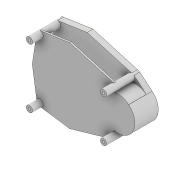
# Autodesk Inventor part: base
Saved by Autodesk Inventor 2020 (Build 240168000, 168)
## iProperties
Created: 2020-08-31
Part Number: base
Material: 일반
Document SubType Name: Modeling
Designer: 이호석
Mass: 51.1495 g
Surface Area: 251.219 cm^2
Volume: 51.1495 cm^3
Density: 1 g/cm^3
Appearance: 기본값
Author: 이호석
Autodesk Inventor part; units mm, degrees
ref_plane "YZ Plane" through (0, 0, 0) normal (1, 0, 0) x (0, 1, 0)
ref_plane "XZ Plane" through (0, 0, 0) normal (0, 1, 0) x (-1, 0, 0)
ref_plane "XY Plane" through (0, 0, 0) normal (0, 0, 1) x (1, 0, 0)
sketch "스케치1" plane through (0, 0, 0) normal (0, 0, 1) x (1, 0, 0)
  line L0 (0, 0) -> (-35.14, 0)
  line L1 (-35.14, 0) -> (61.6, 0)
  line L2 (0, 35.14) -> (0, -35.14)
  line L3 (-35.14, -35.14) -> (61.6, -35.14)
  line L4 (61.6, -35.14) -> (61.6, 35.14)
  line L5 (61.6, 35.14) -> (-35.14, 35.14)
  line L6 (-35.14, 35.14) -> (-35.14, -35.14)
  line L7 (0, 0) -> (-27.87, 0)
  line L8 (0, 0) -> (42, 0)
  line L9 (42, 20) -> (42, -20)
  circle A0 centre (42, -20) radius 1.25
  circle A1 centre (42, 20) radius 1.25
  line L10 (0, 0) -> (45.5, 0)
  circle A2 centre (45.5, 0) radius 9
  circle A3 centre (45.5, 0) radius 16.1
  circle A4 centre (42, -20) radius 3
  circle A5 centre (42, 20) radius 3
  line L11 (45.5, 0) -> (61.6, 0) construction
  line L12 (42, 20) -> (45, 20) construction
  line L13 (44.1213, 22.1213) -> (55.8489, 12.3333)
  line L14 (42, 23) -> (0, 35.14)
  line L15 (-27.87, 28) -> (-27.87, -28)
  circle A6 centre (-27.87, 28) radius 1.25
  circle A7 centre (-27.87, 28) radius 3
  circle A8 centre (-27.87, -28) radius 1.25
  circle A9 centre (-27.87, -28) radius 3
  line L16 (-27.87, 31) -> (0, 35.14)
  line L17 (-30.87, 28) -> (-35.14, 0)
  line L18 (44.1213, -22.1213) -> (55.8489, -12.3333)
  line L19 (42, -23) -> (0, -35.14)
  line L20 (-27.87, -31) -> (0, -35.14)
  line L21 (-30.87, -28) -> (-35.14, 0)
  dimension "d20" = 6
  dimension "d0" = 35.14
  dimension "d1" = 96.74
  dimension "d3" = 70.28
  dimension "d4" = 27.87
  dimension "d9" = 42
  dimension "d11" = 40
  dimension "d12" = 2.5
  dimension "d13" = 2.5
  dimension "d14" = 45.5
  dimension "d15" = 18
  dimension "d16" = 32.2
  dimension "d19" = 6
  dimension "d27" = 56
  dimension "d28" = 2.5
  dimension "d29" = 6
  dimension "d30" = 2.5
  dimension "d31" = 6
  constraints: 44 end point, 10 coincident, 9 centre point, 7 symmetric about line, 5 point on line, 4 horizontal, 4 point on circle, 2 parallel, 1 perpendicular, 3 other
  measures "d0" distance of L0.start L0.end
  measures "d1" distance of L0.end L1.end
  measures "d3" distance of L2.start L2.end
  measures "d4" distance of L0.start L7.end
  measures "d9" distance of L0.start L8.end
  measures "d11" distance of L9.start L9.end
  measures "d12" diameter of A0
  measures "d13" diameter of A1
  measures "d14" distance of L0.start L10.end
  measures "d15" diameter of A2
  measures "d16" diameter of A3
  measures "d19" diameter of A4
  measures "d27" distance of L15.start L15.end
  measures "d28" diameter of A6
  measures "d29" diameter of A7
  measures "d30" diameter of A8
  measures "d31" diameter of A9
extrude "돌출1" add sketch "스케치1" along normal blind 5.5 contours L2 L20 A9 L15 L0 | L2 L14 A5 L9 A3 L1 | L0 L15 A7 L16 L2 | L1 A3 L9 A4 L19 L2 | L15 A9 L21 L0 | L0 L17 A7 L15 | A3 L9 A2 L1 | L1 A2 L9 A3 | A7 | A9 | A2 L9 L1 | L1 L9 A2 | A3 L1 A2 L9 | L9 A5 L13 A3 | A3 L18 A4 L9 | L9 A2 L1 A3 | A5 | A4 | L9 A2 L1 | L1 A2 L9
sketch "스케치2" plane through (0, 0, 5.5) normal (0, 0, 1) x (1, 0, 0)
  line L0 (0, 0) -> (-35.14, 0)
  line L1 (-35.14, 0) -> (61.6, 0)
  line L2 (0, 35.14) -> (0, -35.14)
  line L3 (-35.14, -35.14) -> (61.6, -35.14)
  line L4 (61.6, -35.14) -> (61.6, 35.14)
  line L5 (61.6, 35.14) -> (-35.14, 35.14)
  line L6 (-35.14, 35.14) -> (-35.14, -35.14)
  line L7 (0, 0) -> (-27.87, 0)
  line L8 (0, 0) -> (42, 0)
  line L9 (42, 20) -> (42, -20)
  circle A0 centre (42, -20) radius 1.25
  circle A1 centre (42, 20) radius 1.25
  line L10 (0, 0) -> (45.5, 0)
  circle A2 centre (45.5, 0) radius 9
  circle A3 centre (45.5, 0) radius 16.1
  circle A4 centre (42, -20) radius 3
  circle A5 centre (42, 20) radius 3
  line L11 (45.5, 0) -> (61.6, 0) construction
  line L12 (42, 20) -> (45, 20) construction
  line L13 (44.1213, 22.1213) -> (55.8489, 12.3333)
  line L14 (42, 23) -> (0, 35.14)
  line L15 (-27.87, 28) -> (-27.87, -28)
  circle A6 centre (-27.87, 28) radius 1.25
  circle A7 centre (-27.87, 28) radius 3
  circle A8 centre (-27.87, -28) radius 1.25
  circle A9 centre (-27.87, -28) radius 3
  line L16 (-27.87, 31) -> (0, 35.14)
  line L17 (-30.87, 28) -> (-35.14, 0)
  line L18 (-27.87, -31) -> (0, -35.14)
  line L19 (-30.87, -28) -> (-35.14, 0)
  line L20 (42, -23) -> (0, -35.14)
  line L21 (44.1213, -22.1213) -> (55.8489, -12.3333)
  point P0 (55.7837, -12.3877)
  point P1 (55.7837, 12.3877)
  dimension "d46" = 6
  dimension "d34" = 35.14
  dimension "d35" = 96.74
  dimension "d36" = 70.28
  dimension "d37" = 27.87
  dimension "d38" = 42
  dimension "d39" = 40
  dimension "d40" = 2.5
  dimension "d41" = 2.5
  dimension "d42" = 45.5
  dimension "d43" = 18
  dimension "d44" = 32.2
  dimension "d45" = 6
  dimension "d47" = 56
  dimension "d48" = 2.5
  dimension "d49" = 6
  dimension "d50" = 2.5
  dimension "d51" = 6
  constraints: 44 end point, 10 coincident, 9 centre point, 7 symmetric about line, 5 point on line, 4 horizontal, 4 point on circle, 2 parallel, 1 perpendicular, 1 vertical alignment, 2 other
  measures "d34" distance of L0.start L0.end
  measures "d35" distance of L0.end L1.end
  measures "d36" distance of L2.start L2.end
  measures "d37" distance of L0.start L7.end
  measures "d38" distance of L0.start L8.end
  measures "d39" distance of L9.start L9.end
  measures "d40" diameter of A0
  measures "d41" diameter of A1
  measures "d42" distance of L0.start L10.end
  measures "d43" diameter of A2
  measures "d44" diameter of A3
  measures "d45" diameter of A4
  measures "d47" distance of L15.start L15.end
  measures "d48" diameter of A6
  measures "d49" diameter of A7
  measures "d50" diameter of A8
  measures "d51" diameter of A9
extrude "돌출2" add sketch "스케치2" along normal blind 15 contours A3 L9 A2 L1 | L1 A2 L9 A3 | A7 | A9 | A2 L9 L1 | L1 L9 A2 | A3 L1 A2 L9 | L9 A2 L1 A3 | A5 | A4 | L9 A2 L1 | L1 A2 L9
sketch "스케치3" plane through (0, 0, 20.5) normal (0, 0, 1) x (1, 0, 0)
  line L0 (0, 0) -> (-35.14, 0)
  line L1 (-35.14, 0) -> (61.6, 0)
  line L2 (0, 35.14) -> (0, -35.14)
  line L3 (-35.14, -35.14) -> (61.6, -35.14)
  line L4 (61.6, -35.14) -> (61.6, 35.14)
  line L5 (61.6, 35.14) -> (-35.14, 35.14)
  line L6 (-35.14, 35.14) -> (-35.14, -35.14)
  line L7 (0, 0) -> (-27.87, 0)
  line L8 (0, 0) -> (42, 0)
  line L9 (42, 20) -> (42, -20)
  circle A0 centre (42, -20) radius 1.25
  circle A1 centre (42, 20) radius 1.25
  line L10 (0, 0) -> (45.5, 0)
  circle A2 centre (45.5, 0) radius 9
  circle A3 centre (45.5, 0) radius 16.1
  circle A4 centre (42, -20) radius 3
  circle A5 centre (42, 20) radius 3
  line L11 (45.5, 0) -> (61.6, 0) construction
  line L12 (42, 20) -> (45, 20) construction
  line L13 (44.1213, 22.1213) -> (55.8489, 12.3333)
  line L14 (42, 23) -> (0, 35.14)
  line L15 (-27.87, 28) -> (-27.87, -28)
  circle A6 centre (-27.87, 28) radius 1.25
  circle A7 centre (-27.87, 28) radius 3
  circle A8 centre (-27.87, -28) radius 1.25
  circle A9 centre (-27.87, -28) radius 3
  line L16 (-27.87, 31) -> (0, 35.14)
  line L17 (-30.87, 28) -> (-35.14, 0)
  line L18 (-27.87, -31) -> (0, -35.14)
  line L19 (-30.87, -28) -> (-35.14, 0)
  line L20 (42, -23) -> (0, -35.14)
  line L21 (44.1213, -22.1213) -> (55.8489, -12.3333)
  point P0 (42, -15.715)
  point P1 (55.7837, -12.3877)
  point P2 (55.7837, 12.3877)
  point P3 (42, 15.715)
  point P4 (42, 17)
  point P5 (42, -17)
  dimension "d66" = 6
  dimension "d54" = 35.14
  dimension "d55" = 96.74
  dimension "d56" = 70.28
  dimension "d57" = 27.87
  dimension "d58" = 42
  dimension "d59" = 40
  dimension "d60" = 2.5
  dimension "d61" = 2.5
  dimension "d62" = 45.5
  dimension "d63" = 18
  dimension "d64" = 32.2
  dimension "d65" = 6
  dimension "d67" = 56
  dimension "d68" = 2.5
  dimension "d69" = 6
  dimension "d70" = 2.5
  dimension "d71" = 6
  constraints: 44 end point, 10 coincident, 9 centre point, 7 symmetric about line, 5 point on line, 4 horizontal, 4 point on circle, 2 parallel, 1 perpendicular, 3 other
  measures "d54" distance of L0.start L0.end
  measures "d55" distance of L0.end L1.end
  measures "d56" distance of L2.start L2.end
  measures "d57" distance of L0.start L7.end
  measures "d58" distance of L0.start L8.end
  measures "d59" distance of L9.start L9.end
  measures "d60" diameter of A0
  measures "d61" diameter of A1
  measures "d62" distance of L0.start L10.end
  measures "d63" diameter of A2
  measures "d64" diameter of A3
  measures "d65" diameter of A4
  measures "d67" distance of L15.start L15.end
  measures "d68" diameter of A6
  measures "d69" diameter of A7
  measures "d70" diameter of A8
  measures "d71" diameter of A9
extrude "돌출3" add sketch "스케치3" along normal blind 1.6 contours L2 L18 A9 L15 L0 | L2 L14 A5 L9 A3 L1 | L0 L15 A7 L16 L2 | L1 A3 L9 A4 L20 L2 | L15 A9 L19 L0 | L0 L17 A7 L15 | A3 L9 A2 L1 | L1 A2 L9 A3 | A7 | A9 | A2 L9 L1 | L1 L9 A2 | A3 L1 A2 L9 | L9 A2 L1 A3 | A5 | A4 | L9 A2 L1 | L1 A2 L9
sketch "스케치4" plane through (0, 0, 22.1) normal (0, 0, 1) x (1, 0, 0)
  line L0 (0, 0) -> (-35.14, 0)
  line L1 (-35.14, 0) -> (61.6, 0)
  line L2 (0, 35.14) -> (0, -35.14)
  line L3 (-35.14, -35.14) -> (61.6, -35.14)
  line L4 (61.6, -35.14) -> (61.6, 35.14)
  line L5 (61.6, 35.14) -> (-35.14, 35.14)
  line L6 (-35.14, 35.14) -> (-35.14, -35.14)
  line L7 (0, 0) -> (-27.87, 0)
  line L8 (0, 0) -> (42, 0)
  line L9 (42, 20) -> (42, -20)
  circle A0 centre (42, -20) radius 1.25
  circle A1 centre (42, 20) radius 1.25
  line L10 (0, 0) -> (45.5, 0)
  circle A2 centre (45.5, 0) radius 9
  circle A3 centre (45.5, 0) radius 16.1
  circle A4 centre (42, -20) radius 3
  circle A5 centre (42, 20) radius 3
  line L11 (45.5, 0) -> (61.6, 0) construction
  line L12 (42, 20) -> (45, 20) construction
  line L13 (44.1213, 22.1213) -> (55.8489, 12.3333)
  line L14 (42, 23) -> (0, 35.14)
  line L15 (-27.87, 28) -> (-27.87, -28)
  circle A6 centre (-27.87, 28) radius 1.25
  circle A7 centre (-27.87, 28) radius 3
  circle A8 centre (-27.87, -28) radius 1.25
  circle A9 centre (-27.87, -28) radius 3
  line L16 (-27.87, 31) -> (0, 35.14)
  line L17 (-30.87, 28) -> (-35.14, 0)
  line L18 (-27.87, -31) -> (0, -35.14)
  line L19 (-30.87, -28) -> (-35.14, 0)
  line L20 (42, -23) -> (0, -35.14)
  line L21 (44.1213, -22.1213) -> (55.8489, -12.3333)
  dimension "d86" = 6
  dimension "d74" = 35.14
  dimension "d75" = 96.74
  dimension "d76" = 70.28
  dimension "d77" = 27.87
  dimension "d78" = 42
  dimension "d79" = 40
  dimension "d80" = 2.5
  dimension "d81" = 2.5
  dimension "d82" = 45.5
  dimension "d83" = 18
  dimension "d84" = 32.2
  dimension "d85" = 6
  dimension "d87" = 56
  dimension "d88" = 2.5
  dimension "d89" = 6
  dimension "d90" = 2.5
  dimension "d91" = 6
  constraints: 44 end point, 10 coincident, 9 centre point, 7 symmetric about line, 5 point on line, 4 horizontal, 4 point on circle, 2 parallel, 1 perpendicular, 1 vertical alignment, 2 other
  measures "d74" distance of L0.start L0.end
  measures "d75" distance of L0.end L1.end
  measures "d76" distance of L2.start L2.end
  measures "d77" distance of L0.start L7.end
  measures "d78" distance of L0.start L8.end
  measures "d79" distance of L9.start L9.end
  measures "d80" diameter of A0
  measures "d81" diameter of A1
  measures "d82" distance of L0.start L10.end
  measures "d83" diameter of A2
  measures "d84" diameter of A3
  measures "d85" diameter of A4
  measures "d87" distance of L15.start L15.end
  measures "d88" diameter of A6
  measures "d89" diameter of A7
  measures "d90" diameter of A8
  measures "d91" diameter of A9
extrude "돌출4" add sketch "스케치4" along normal blind 10 contours A7 | A9 | A5 | A4
